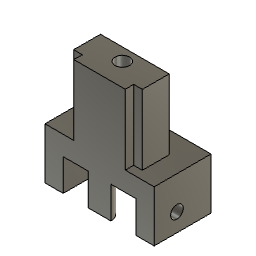
tip_holder_puzzle (Autodesk Fusion 360 design; units mm, degrees)
Autodesk Fusion 360 part; units mm, degrees
sketch "Sketch1" plane through (0, 0, 0) normal (0, 0, 1) x (1, 0, 0)
  line L0 (0, 0) -> (26.67, 0)
  line L1 (26.67, 0) -> (26.67, 12.7)
  line L2 (26.67, 12.7) -> (0, 12.7)
  line L3 (0, 12.7) -> (0, 0)
  line L4 (0, 0) -> (3.175, 0)
  line L5 (3.175, 0) -> (3.175, 12.7)
  line L6 (3.175, 12.7) -> (0, 12.7)
  line L7 (0, 12.7) -> (0, 0)
  line L8 (26.67, 0) -> (23.495, 0)
  line L9 (23.495, 0) -> (23.495, 12.7)
  line L10 (23.495, 12.7) -> (26.67, 12.7)
  line L11 (26.67, 12.7) -> (26.67, 0)
  circle A0 centre (13.335, 6.35) radius 2.05
  line L12 (13.335, 12.7) -> (13.335, 0) construction
  line L13 (3.175, 6.35) -> (23.495, 6.35) construction
  point P0 (13.335, 6.35)
  dimension "d1" = 26.67
  dimension "d2" = 12.7
  dimension "d3" = 3.175
  dimension "d4" = 3.175
  dimension "d5" = 4.1
  constraint horizontal L0
  constraint vertical L1
  constraint horizontal L2
  constraint vertical L3
  constraint coincident L0.start L3.end
  constraint horizontal L4
  constraint vertical L5
  constraint horizontal L6
  constraint vertical L7
  constraint horizontal L8
  constraint vertical L9
  constraint horizontal L10
  constraint vertical L11
  constraint midpoint L2 L12.start
  constraint midpoint L0 L12.end
  constraint midpoint L5 L13.start
  constraint midpoint L9 L13.end
  constraint midpoint L13 P0
  measures "d1" distance of L0.start L0.end
  measures "d2" distance of L0.start L2.end
  measures "d3" distance of L0.start L4.end
  measures "d4" distance of L0.end L8.end
  measures "d5" diameter of A0
extrude "Extrude1" add sketch "Sketch1" along normal blind 5.4
extrude "Extrude3" add sketch "Sketch1" against normal blind 7.62 contours L0 L1 L2 L8 L9 L10 L11
extrude "Extrude4" add sketch "Sketch1" against normal blind 8.89 contours L0 L2 L3 L4 L5 L6 L7
ref_plane "WorkPlane1" through (13.335, 6.35, 2.21) normal (0, 0, 1) x (1, 0, 0)
sketch "Sketch2" plane through (0, 0, 2.21) normal (0, 0, 1) x (1, 0, 0)
  circle A0 centre (13.3518, 6.366) radius 2.05
  dimension "d15" = 4.1
  measures "d15" diameter of A0
sketch "Sketch3" plane through (0, 0, 0) normal (0, 0, 1) x (1, 0, 0)
  circle A0 centre (13.335, 6.35) radius 4
  circle A1 centre (13.335, 6.35) radius 2.05
  dimension "d16" = 8
  constraint concentric A0 A1
  measures "d16" diameter of A0
loft "Loft1" cut profiles "Sketch3", "Sketch2" section 1 section 2
sketch "Sketch4" plane through (23.495, 0, 0) normal (-1, 0, 0) x (0, -1, 0)
  line L0 (0, 0) -> (-12.7, 0)
  line L1 (-12.7, 0) -> (-12.7, -7.62)
  line L2 (-12.7, -7.62) -> (0, -7.62)
  line L3 (0, -7.62) -> (0, 0)
  circle A0 centre (-6.35, -3.81) radius 1.778
  dimension "d17" = 3.556
  measures "d17" diameter of A0
extrude "Extrude5" cut sketch "Sketch4" along normal blind 26 and the other way blind 17 contours A0
sketch "Sketch5" plane through (0, 0, 5.4) normal (0, 0, 1) x (-1, 0, 0)
  circle A0 centre (-13.335, -6.35) radius 2.05
  line L0 (-26.67, -12.7) -> (0, -12.7)
  line L1 (0, -12.7) -> (0, 0)
  line L2 (0, 0) -> (-26.67, 0)
  line L3 (-26.67, 0) -> (-26.67, -12.7)
  line L4 (-13.335, 0) -> (-13.335, -12.7) construction
  line L5 (0, -6.35) -> (-26.67, -6.35) construction
  line L6 (-6.1595, -2.3495) -> (-20.5105, -2.3495)
  line L7 (-20.5105, -2.3495) -> (-20.5105, -10.3505)
  line L8 (-20.5105, -10.3505) -> (-6.1595, -10.3505)
  line L9 (-6.1595, -10.3505) -> (-6.1595, -2.3495)
  line L10 (-6.1595, -2.3495) -> (-20.5105, -10.3505) construction
  line L11 (-20.5105, -2.3495) -> (-6.1595, -10.3505) construction
  line L12 (-20.5105, -2.3495) -> (-6.1595, -2.3495)
  point P0 (-13.335, -6.35)
  point P1 (-13.335, -6.35)
  dimension "d26" = 14.351
  dimension "d27" = 8.001
  dimension "d28" = 14.351
  constraint midpoint L2 L4.start
  constraint midpoint L0 L4.end
  constraint midpoint L1 L5.start
  constraint midpoint L3 L5.end
  constraint coincident P0 A0.centre
  constraint horizontal L6
  constraint perpendicular L6 L7
  constraint parallel L6 L8
  constraint parallel L7 L9
  constraint coincident L10 P1
  constraint coincident L11 P1
  constraint horizontal L12
  measures "d26" distance of L7.end L8.end
  measures "d27" distance of L6.end L7.end
  measures "d28" distance of L6.end L6.start
extrude "Extrude6" add sketch "Sketch5" along normal blind 8.128 contours L6 L7 L8 L9 L12
sketch "Sketch6" plane through (0, 0, 13.528) normal (0, 0, 1) x (-1, 0, 0)
  circle A0 centre (-13.335, -6.35) radius 2.05
  line L0 (-6.1595, -2.3495) -> (-20.5105, -2.3495)
  line L1 (-20.5105, -2.3495) -> (-20.5105, -10.3505)
  line L2 (-20.5105, -10.3505) -> (-6.1595, -10.3505)
  line L3 (-6.1595, -10.3505) -> (-6.1595, -2.3495)
  line L4 (-20.5105, -2.3495) -> (-6.1595, -2.3495)
  line L5 (-6.1595, -2.3495) -> (-6.1595, 0.9525)
  line L6 (-6.1595, 0.9525) -> (-20.5105, 0.9525)
  line L7 (-20.5105, 0.9525) -> (-20.5105, -2.3495)
  line L8 (-3.7465, -2.3495) -> (-22.9235, -2.3495)
  line L9 (-22.9235, -2.3495) -> (-22.9235, -10.3505)
  line L10 (-22.9235, -10.3505) -> (-3.7465, -10.3505)
  line L11 (-3.7465, -10.3505) -> (-3.7465, -2.3495)
  line L12 (-3.7465, -2.3495) -> (-22.9235, -10.3505) construction
  line L13 (-22.9235, -2.3495) -> (-3.7465, -10.3505) construction
  point P0 (-13.335, -6.35)
  dimension "d30" = 14.351
  dimension "d31" = 3.302
  dimension "d32" = 19.177
  dimension "d33" = 8.001
  constraint horizontal L4
  constraint vertical L5
  constraint horizontal L6
  constraint vertical L7
  constraint coincident L0.end L1.start
  constraint horizontal L8
  constraint perpendicular L8 L9
  constraint parallel L8 L10
  constraint parallel L9 L11
  constraint coincident L12 P0
  constraint coincident L13 P0
  constraint coincident P0 A0.centre
  measures "d30" distance of L0.end L0.start
  measures "d31" distance of L0.end L6.end
  measures "d32" distance of L9.end L10.end
  measures "d33" distance of L8.end L9.end
extrude "Extrude7" add sketch "Sketch6" along normal blind -3.175 and the other way blind -11.43
sketch "Sketch7" plane through (0, 0, 24.958) normal (0, 0, 1) x (-1, 0, 0)
  circle A0 centre (-13.335, -6.35) radius 2.05
  line L0 (-22.9235, -10.3505) -> (-3.7465, -10.3505)
  line L1 (-3.7465, -10.3505) -> (-3.7465, -2.3495)
  line L2 (-3.7465, -2.3495) -> (-6.1595, -2.3495)
  line L3 (-6.1595, -2.3495) -> (-6.1595, 0.9525)
  line L4 (-6.1595, 0.9525) -> (-20.5105, 0.9525)
  line L5 (-20.5105, 0.9525) -> (-20.5105, -2.3495)
  line L6 (-20.5105, -2.3495) -> (-22.9235, -2.3495)
  line L7 (-22.9235, -2.3495) -> (-22.9235, -10.3505)
  line L8 (-13.335, -6.35) -> (-7.5565, -6.35) construction
  line L9 (-13.335, -6.35) -> (-9.3345, -6.35) construction
  line L10 (-17.3355, -2.3495) -> (-9.3345, -2.3495)
  line L11 (-9.3345, -6.35) -> (-9.3345, -2.3495) construction
  line L12 (-9.3345, -6.35) -> (-9.3345, -10.3505) construction
  arc A1 (-9.3345, -10.3505) -> (-9.3345, -2.3495) centre (-12.9461, -6.35) ccw
  line L13 (-13.335, -6.35) -> (-19.1135, -6.35) construction
  line L14 (-13.335, -6.35) -> (-17.3355, -6.35) construction
  line L15 (-17.3355, -6.35) -> (-17.3355, -2.3495) construction
  line L16 (-17.3355, -6.35) -> (-17.3355, -10.3505) construction
  arc A2 (-17.3355, -2.3495) -> (-17.3355, -10.3505) centre (-13.7239, -6.35) ccw
  dimension "d36" = 5.7785
  dimension "d37" = 4.0005
  dimension "d38" = 5.7785
  dimension "d39" = 4.0005
  constraint coincident A0.centre L8.start
  constraint horizontal L8
  constraint parallel L8 L9
  constraint perpendicular L10 L11
  constraint coincident L0 L12.end
  constraint perpendicular L0 L12
  constraint coincident L8.end A1
  constraint parallel L8 L13
  constraint parallel L13 L14
  constraint perpendicular L10 L15
  constraint coincident L0 L16.end
  constraint perpendicular L0 L16
  constraint coincident L13.end A2
  measures "d36" distance of A0.centre L8.end
  measures "d37" distance of A0.centre L9.end
  measures "d38" distance of A0.centre L13.end
  measures "d39" distance of A0.centre L14.end
sketch "Sketch9" plane through (0, 10.3505, 0) normal (0, 1, 0) x (-1, 0, 0)
  line L0 (-20.5105, 10.353) -> (-20.5105, 5.4)
  line L1 (-20.5105, 5.4) -> (-6.1595, 5.4)
  line L2 (-6.1595, 5.4) -> (-6.1595, 10.353)
  line L3 (-6.1595, 10.353) -> (-3.7465, 10.353)
  line L4 (-3.7465, 10.353) -> (-3.7465, 24.958)
  line L5 (-3.7465, 24.958) -> (-22.9235, 24.958)
  line L6 (-22.9235, 24.958) -> (-22.9235, 10.353)
  line L7 (-22.9235, 10.353) -> (-20.5105, 10.353)
  line L8 (-17.3355, 14.4805) -> (-9.3345, 14.4805)
  line L9 (-9.3345, 20.8305) -> (-17.3355, 20.8305)
  arc A0 (-9.3345, 14.4805) -> (-9.3345, 20.8305) centre (-19.0024, 17.6555) ccw
  arc A1 (-17.3355, 20.8305) -> (-17.3355, 14.4805) centre (-7.6676, 17.6555) ccw
  line L10 (-17.8435, 15.494) -> (-17.6113, 15.494) construction
  line L11 (-13.335, 24.958) -> (-13.335, 20.8305) construction
  line L12 (-13.335, 14.4805) -> (-13.335, 10.16) construction
  line L13 (-22.9235, 17.6555) -> (-17.8435, 17.6555) construction
  line L14 (-8.8265, 17.6555) -> (-3.7465, 17.6555) construction
  line L15 (-20.5105, 10.353) -> (-20.5105, 5.4)
  line L16 (-20.5105, 5.4) -> (-6.1595, 5.4)
  line L17 (-6.1595, 5.4) -> (-6.1595, 10.353)
  line L18 (-6.1595, 10.353) -> (-3.7465, 10.353)
  line L19 (-3.7465, 10.353) -> (-3.7465, 24.958)
  line L20 (-3.7465, 24.958) -> (-22.9235, 24.958)
  line L21 (-22.9235, 24.958) -> (-22.9235, 10.353)
  line L22 (-22.9235, 10.353) -> (-20.5105, 10.353)
  line L23 (-6.1595, 24.958) -> (-6.1595, 10.353)
  line L24 (-6.1595, 10.353) -> (-20.5105, 10.353)
  line L25 (-20.5105, 10.353) -> (-20.5105, 24.958)
  line L26 (-20.5105, 24.958) -> (-6.1595, 24.958)
  line L27 (-20.5105, 10.353) -> (-20.5105, 5.4)
  line L28 (-20.5105, 5.4) -> (-6.1595, 5.4)
  line L29 (-6.1595, 5.4) -> (-6.1595, 10.353)
  line L30 (-6.1595, 10.353) -> (-3.7465, 10.353)
  line L31 (-3.7465, 10.353) -> (-3.7465, 24.958)
  line L32 (-3.7465, 24.958) -> (-22.9235, 24.958)
  line L33 (-22.9235, 24.958) -> (-22.9235, 10.353)
  line L34 (-22.9235, 10.353) -> (-20.5105, 10.353)
  point P0 (-13.335, 17.6555)
  dimension "d56" = 8.001
  dimension "d57" = 6.35
  constraint midpoint L6 L13.start
  constraint midpoint L4 L14.end
  constraint midpoint L5 L11.start
  constraint perpendicular L11 L13
  constraint horizontal L8
  constraint parallel L8 L9
  constraint horizontal L10
  constraint coincident A1 L10.end
  constraint collinear L11 L12
  constraint coincident L8 L12.start
  constraint coincident A1 L13.end
  constraint coincident A0 L14.start
  constraint collinear L13 L14
  constraint coincident L9 L11.end
  measures "d56" distance of L9.start L9.end
  measures "d57" distance of L8.end L9.start
extrude "Extrude11" cut sketch "Sketch9" against normal blind 8.001 contours L8 L9 A0 A1
extrude "Extrude12" add 3 faces at (10.9432, 1.2488, 10.353) (4.5508, 7.6835, 10.353) (21.3148, 7.6835, 10.353) along direction (0, 0, -1) blind 4.953
extrude "Extrude13" add 1 faces at (26.67, 6.3943, 2.921) along direction (1, 0, 0) blind 1.905
extrude "Extrude14" add 1 faces at (0, 6.3057, 2.921) along direction (-1, 0, 0) blind 1.905
sketch "Sketch10" plane through (0, 0, 0) normal (0, 0, -1) x (1, 0, 0)
  circle A0 centre (13.335, -6.35) radius 4
  line L0 (3.175, 0) -> (3.175, -12.7)
  line L1 (3.175, -12.7) -> (23.495, -12.7)
  line L2 (23.495, -12.7) -> (23.495, 0)
  line L3 (23.495, 0) -> (3.175, 0)
  circle A1 centre (13.335, 0) radius 3.175
  dimension "d69" = 6.35
  constraint midpoint L3 A1.centre
  measures "d69" diameter of A1
extrude "Extrude15" cut 1 faces at (10.9432, -0.3175, 5.4) along direction (0, 0, 1) blind 26.67
extrude "Extrude16" add sketch "Sketch10" along normal up to surface (8.89 mm away) contours A0 A1 | A0 L3 A1 picked at (13.6688, -2.6285)
extrude "Extrude17" add 1 faces at (16.7217, 12.7, 3.6) along direction (0, 1, 0) blind 3.175
sketch "Sketch11" plane through (0, 0, 0) normal (0, 0, -1) x (1, 0, 0)
  arc A0 (14.991, -2.7089) -> (16.51, 0) centre (13.335, 0) ccw
  arc A1 (11.679, -2.7089) -> (14.991, -2.7089) centre (13.335, -6.35) ccw
  arc A2 (10.16, 0) -> (11.679, -2.7089) centre (13.335, 0) ccw
  line L0 (10.16, 0) -> (3.175, 0)
  line L1 (3.175, 0) -> (3.175, -15.875)
  line L2 (3.175, -15.875) -> (23.495, -15.875)
  line L3 (23.495, -15.875) -> (23.495, 0)
  line L4 (23.495, 0) -> (16.51, 0)
  line L5 (3.175, -15.875) -> (8.255, -15.875)
  line L6 (8.255, -15.875) -> (8.255, -12.7)
  line L7 (8.255, -12.7) -> (3.175, -12.7)
  line L8 (3.175, -12.7) -> (3.175, -15.875)
  line L9 (23.495, -15.875) -> (18.415, -15.875)
  line L10 (18.415, -15.875) -> (18.415, -12.7)
  line L11 (18.415, -12.7) -> (23.495, -12.7)
  line L12 (23.495, -12.7) -> (23.495, -15.875)
  dimension "d74" = 5.08
  dimension "d75" = 3.175
  dimension "d76" = 5.08
  dimension "d77" = 3.175
  constraint horizontal L5
  constraint vertical L6
  constraint horizontal L7
  constraint vertical L8
  constraint coincident L1.end L2.start
  constraint horizontal L9
  constraint vertical L10
  constraint horizontal L11
  constraint vertical L12
  constraint coincident L2.end L3.start
  measures "d74" distance of L1.end L5.end
  measures "d75" distance of L1.end L7.end
  measures "d76" distance of L2.end L9.end
  measures "d77" distance of L2.end L11.end
extrude "Extrude18" add sketch "Sketch11" along normal up to surface (8.89 mm away) contours L2 L3 L9 L10 L11 L12 | L1 L2 L5 L6 L7 L8
sketch "Sketch12" plane through (0, 0, 0) normal (0, 0, -1) x (1, 0, 0)
  line L0 (3.175, -12.7) -> (8.255, -12.7)
  line L1 (8.255, -12.7) -> (8.255, -15.875)
  line L2 (8.255, -15.875) -> (18.415, -15.875)
  line L3 (18.415, -15.875) -> (18.415, -12.7)
  line L4 (18.415, -12.7) -> (23.495, -12.7)
  line L5 (23.495, -12.7) -> (23.495, 0)
  line L6 (23.495, 0) -> (16.51, 0)
  arc A0 (14.991, -2.7089) -> (16.51, 0) centre (13.335, 0) ccw
  arc A1 (11.679, -2.7089) -> (14.991, -2.7089) centre (13.335, -6.35) ccw
  arc A2 (10.16, 0) -> (11.679, -2.7089) centre (13.335, 0) ccw
  line L7 (10.16, 0) -> (3.175, 0)
  line L8 (3.175, 0) -> (3.175, -12.7)
  circle A3 centre (13.335, -6.35) radius 4
  constraint concentric A1 A3
extrude "Extrude19" cut sketch "Sketch12" along normal blind 20.32 contours A1 A3
sketch "Sketch13" plane through (0, 0, 24.958) normal (0, 0, 1) x (-1, 0, 0)
  line L0 (-6.1595, 0) -> (-20.5105, 0)
  line L1 (-20.5105, 0) -> (-20.5105, -2.3495)
  line L2 (-20.5105, -2.3495) -> (-22.9235, -2.3495)
  line L3 (-22.9235, -2.3495) -> (-22.9235, -10.3505)
  line L4 (-22.9235, -10.3505) -> (-3.7465, -10.3505)
  line L5 (-3.7465, -10.3505) -> (-3.7465, -2.3495)
  line L6 (-3.7465, -2.3495) -> (-6.1595, -2.3495)
  line L7 (-6.1595, -2.3495) -> (-6.1595, 0)
  circle A0 centre (-13.335, -6.35) radius 2.05
  line L8 (-3.7465, -10.3505) -> (-22.9235, -10.3505)
  line L9 (-22.9235, -10.3505) -> (-22.9235, -9.8425)
  line L10 (-22.9235, -9.8425) -> (-3.7465, -9.8425)
  line L11 (-3.7465, -9.8425) -> (-3.7465, -10.3505)
  dimension "d82" = 0.508
  constraint horizontal L8
  constraint vertical L9
  constraint horizontal L10
  constraint vertical L11
  constraint coincident L4.end L5.start
  measures "d82" distance of L4.end L10.end
extrude "Extrude20" cut sketch "Sketch13" against normal up to surface (19.558 mm away) contours L3 L4 L5 L8 L9 L10 L11
extrude "Extrude21" add 1 faces at (26.8817, 9.525, -7.62) along direction (0, 0, -1) up to surface (1.27 mm away)
